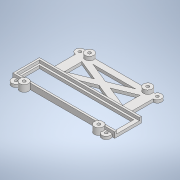
# Autodesk Inventor part: top_v2
Saved by Autodesk Inventor 2020.4 (Build 244396000, 396)
## iProperties
Created: 2021-05-30
Part Number: top_v2
Material: Generic
Document SubType Name: Modeling
Designer: Tarsoly
Density: 1 g/cm^3
Appearance: Default
Author: Tarsoly
Autodesk Inventor part; units mm, degrees
ref_plane "YZ Plane" through (0, 0, 0) normal (1, 0, 0) x (0, 1, 0)
ref_plane "XZ Plane" through (0, 0, 0) normal (0, 1, 0) x (-1, 0, 0)
ref_plane "XY Plane" through (0, 0, 0) normal (0, 0, 1) x (1, 0, 0)
sketch "Sketch1" plane through (0, 0, 0) normal (0, 1, 0) x (-1, 0, 0)
  line L0 (-51.5, 20.6188) -> (51.5, 20.6188) construction
  line L1 (51.5, 20.6188) -> (51.5, -3.3812) construction
  line L2 (-51.5, -3.3812) -> (51.5, -3.3812) construction
  line L3 (-51.5, 20.6188) -> (-51.5, -3.3812) construction
  circle A0 centre (-40.639, -35.0012) radius 1.5 projected
  circle A1 centre (-46.9907, 24.9986) radius 1.5 projected
  circle A2 centre (47.7513, 25.0014) radius 1.5 projected
  circle A3 centre (40.641, -34.9988) radius 1.5 projected
  circle A4 centre (30.6145, -35) radius 1.6 projected
  circle A5 centre (-30.6145, -35) radius 1.6 projected
  circle A6 centre (-39.2078, 25) radius 1.7 projected
  circle A7 centre (39.2078, 25) radius 1.6 projected
  line L4 (49.5, -1.3812) -> (49.5, 18.6188)
  line L5 (49.5, 18.6188) -> (-49.5, 18.6188)
  line L6 (-49.5, 18.6188) -> (-49.5, -1.3812)
  line L7 (-49.5, -1.3812) -> (49.5, -1.3812)
  line L8 (53.5, -5.3812) -> (53.5, 22.6188)
  line L9 (53.5, 22.6188) -> (-53.5, 22.6188)
  line L10 (-53.5, 22.6188) -> (-53.5, -5.3812)
  line L11 (-53.5, -5.3812) -> (53.5, -5.3812)
  circle A8 centre (-40.639, -35.0012) radius 4.5
  circle A9 centre (-30.6145, -35) radius 4.6
  circle A10 centre (30.6145, -35) radius 4.6
  circle A11 centre (40.641, -34.9988) radius 4.5
  circle A12 centre (39.2078, 25) radius 4.6
  circle A13 centre (47.7513, 25.0014) radius 4.5
  circle A14 centre (-39.2078, 25) radius 4.7
  circle A15 centre (-46.9907, 24.9986) radius 4.5
  line L12 (-40.6538, -36.5011) -> (-30.6303, -36.5999)
  line L13 (-30.6145, -33.4) -> (-30.6145, -5.3812)
  line L14 (-40.639, -33.5012) -> (-40.639, -5.3812)
  line L15 (40.6561, -36.4987) -> (30.6303, -36.5999)
  line L16 (30.6145, -33.4) -> (30.6145, -5.3812)
  line L17 (40.641, -33.4988) -> (40.641, -5.3812)
  line L18 (-30.6303, -36.5999) -> (30.6303, -36.5999)
  line L19 (-30.6145, -30.4) -> (30.6145, -30.4)
  line L20 (-30.6145, -27.0512) -> (22.419, -5.3812)
  line L21 (-22.419, -30.4) -> (30.6145, -8.73)
  line L22 (22.419, -30.4) -> (-30.6145, -8.73)
  line L23 (-22.419, -5.3812) -> (30.6145, -27.0512)
  line L24 (-30.6145, -5.3812) -> (30.6145, -30.4) construction
  line L25 (30.6145, -5.3812) -> (-30.6145, -30.4) construction
  point P0 (0, 0)
  point P1 (42.2596, 13.6212)
  point P2 (35.2721, 22.6188)
  point P3 (-35.1556, 22.6188)
  point P4 (-43.2179, 27.4513)
  point P5 (-50.8099, 22.6188)
  point P6 (-40.639, -30.5012)
  point P7 (-36.4113, -36.5429)
  point P8 (-34.9429, -36.5574)
  point P9 (-26.3017, -36.5999)
  point P10 (26.3017, -36.5999)
  point P11 (34.9432, -36.5564)
  point P12 (36.4137, -36.5416)
  point P13 (40.641, -30.4988)
  point P14 (51.5688, 22.6188)
  point P15 (43.5325, 26.5673)
  point P16 (8.1955, -17.8906)
  point P17 (0, -14.5418)
  point P18 (-8.1955, -17.8906)
  point P19 (0, -21.2394)
  point P20 (-30.5988, -36.5999)
  point P21 (-43.2599, 22.6188)
  point P22 (-43.1715, 22.6188)
  point P23 (-43.217, 22.5473)
  point P24 (43.1435, 22.6188)
  point P25 (43.533, 23.4341)
  point P26 (43.9338, 22.6188)
  dimension "d0" = 2
  dimension "d1" = 2
  dimension "d2" = 3
  dimension "d3" = 3
  dimension "d4" = 3
  dimension "d5" = 3
  dimension "d6" = 3
  dimension "d7" = 3
  dimension "d8" = 3
  dimension "d9" = 3
  dimension "d10" = 6.1999
  dimension "d11" = 6.1999
  dimension "d12" = 6.1999
  dimension "d13" = 3.1
  dimension "d14" = 3.1
  constraints: 44 end point, 18 point on line, 8 point on circle, 6 centre point, 4 parallel, 4 perpendicular, 4 tangent, 1 horizontal, 13 other
  measures "d0" distance between parallel lines of L2 L7
  measures "d1" distance between parallel lines of L2 L11
  measures "d2" radial gap between concentric circles of A0 A8
  measures "d5" radial gap between concentric circles of A3 A11
  measures "d6" radial gap between concentric circles of A7 A12
  measures "d7" radial gap between concentric circles of A2 A13
  measures "d8" radial gap between concentric circles of A6 A14
  measures "d9" radial gap between concentric circles of A1 A15
  measures "d10" vertical distance of L19.end L15.end
  measures "d11" distance between parallel lines of L20 L21
  measures "d12" distance between parallel lines of L23 L22
  measures "d13" distance between parallel lines of L25 L21
  measures "d14" distance between parallel lines of L24 L22
extrude "Extrusion1" add sketch "Sketch1" against normal blind 3 contours A0 L14 A8 L12 | A0 L12 A8 L14 | L14 L11 L13 A9 L12 A8 | L11 L10 L9 A15 A14 A12 A13 L8 | L12 L18 A9 | A9 L13 A5 L12 | L11 L23 L20 L22 L13 | L19 A10 L18 A9 | A9 L18 A5 L13 | L13 L20 L22 L21 L19 | A10 L16 A4 L15 | A15 A14 L9 | L9 A14 A15 | L11 L16 L21 L23 L20 | L23 L21 L22 L20 | L22 L21 L23 L16 L19 | L16 L11 L17 A11 L15 A10 | A10 L15 A4 L16 | A14 A15 L9 | A14 L9 A15 | A15 L9 A14 | L15 A3 L17 A11 | A11 L17 A3 L15 | A12 A13 L9 | L9 A12 | A13 L9 A12 | A12 A13 | L9 A13 picked at (-47.0805, 22.9157) picked at (-48.0862, 22.3567) picked at (-43.4171, 25.0266) picked at (-39.11, 22.85) picked at (-38.0431, 22.3329) picked at (39.2721, 22.8831) picked at (47.691, 22.9166)
sketch "Sketch2" plane through (0, 0, 0) normal (0, 1, 0) x (1, 0, 0)
  line L0 (-51.5, -20.6188) -> (51.5, -20.6188) projected
  line L1 (51.5, -20.6188) -> (51.5, 3.3812) projected
  line L2 (-51.5, 3.3812) -> (51.5, 3.3812) projected
  line L3 (-51.5, -20.6188) -> (-51.5, 3.3812) projected
  line L4 (-51.5, -20.6188) -> (51.5, -20.6188) projected
  line L5 (8, -22.6188) -> (36.5703, -22.6188) projected
  line L6 (-53.5, 5.3812) -> (-53.5, -22.6188) projected
  line L7 (-53.5, 5.3812) -> (53.5, 5.3812)
  line L8 (53.5, 5.3812) -> (53.5, -22.6188)
  line L9 (53.5, -22.6188) -> (-53.5, -22.6188)
  line L10 (-53.5, -22.6188) -> (-53.5, 5.3812)
  line L11 (51.5, 3.3812) -> (53.5, 3.3812)
  line L12 (53.5, 5.3812) -> (53.5, -22.6188) projected
  line L13 (51.5, -20.6188) -> (53.5, -20.6188)
  constraints: 12 end point, 3 parallel, 2 perpendicular, 2 point on line, 1 horizontal, 2 other
extrude "Extrusion2" add sketch "Sketch2" along normal blind 3 contours L0 L13 L8 L9 L5 L6 L7 L11 L2 L3
sketch "Sketch3" plane through (0, 0, 0) normal (0, 1, 0) x (1, 0, 0)
  arc A0 (34.9429, 36.5574) -> (26.3017, 36.5999) centre (30.6145, 35) ccw projected
  arc A1 (-26.3017, 36.5999) -> (-34.9432, 36.5564) centre (-30.6145, 35) ccw projected
  arc A2 (-43.5325, -26.5673) -> (-35.2721, -22.6188) centre (-39.2078, -25) ccw projected
  arc A3 (35.1556, -22.6188) -> (43.2179, -27.4513) centre (39.2078, -25) ccw projected
  circle A4 centre (-30.6145, 35) radius 1.6 projected
  circle A5 centre (-39.2078, -25) radius 1.6 projected
  circle A6 centre (39.2078, -25) radius 1.6 projected
  circle A7 centre (30.6145, 35) radius 1.6 projected
  circle A8 centre (30.6145, 35) radius 4.6
  circle A9 centre (39.2078, -25) radius 4.7
  circle A10 centre (-39.2078, -25) radius 1.6 projected
  circle A11 centre (-39.2078, -25) radius 4.6
  circle A12 centre (-30.6145, 35) radius 4.6
  line L0 (-51.5, -20.6188) -> (51.5, -20.6188) projected
  line L1 (-51.5, -20.6188) -> (51.5, -20.6188) projected
  point P0 (0, 0)
  point P1 (-37.806, -20.6188)
  point P2 (-40.6096, -20.6188)
  point P3 (40.9093, -20.6188)
  point P4 (37.5063, -20.6188)
  point P5 (43.2179, -27.4513)
  constraints: 4 centre point, 4 coincident, 4 concentric
extrude "Extrusion3" add sketch "Sketch3" along normal blind 4 contours A8 A0 | A12 A1 | A11 L0 A2 | A9 L0 A3
equation "\"d11\" = d10"
equation "\"d12\" = d10"
equation "\"d13\" = 0.5 * d11"
equation "\"d14\" = 0.5 * d12"
equation "\"d15\" = d3"
body "Solid1"
